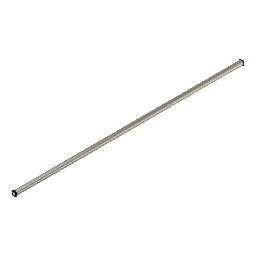
Linear_rail_X_F01 (Autodesk Fusion 360 design; units mm, degrees)
Autodesk Fusion 360 part; units mm, degrees
cylinder "円柱プリミティブ1" add diameter 8 height 370 placed x (1, 0, 0) y (0, 0, -1) z (0, 1, 0) at (0, 0, 0)
chamfer "面取り1" distance 1 angle 45 2 edges at (-3.7293, 370, 1.4465) (-3.7293, 0, -1.4465)
